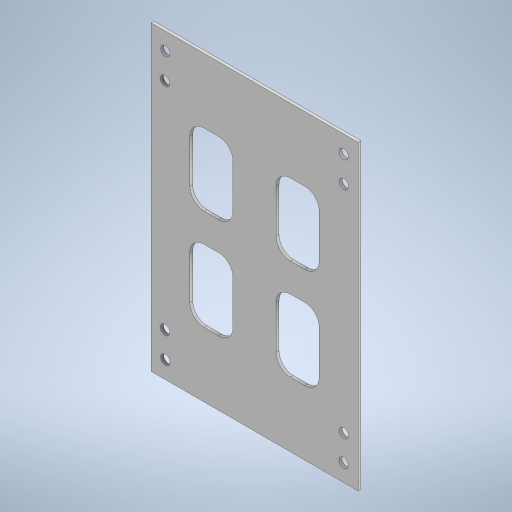
# Autodesk Inventor part: battery_box_24V_side1
Saved by Autodesk Inventor 2023 (Build 270158000, 158)
## iProperties
Created: 2023-05-28
Part Number: battery_box_24V_side1
Material: 一般
Document SubType Name: Sheet Metal
Designer: 310611102
Density: 1 g/cm^3
Sheet Metal Rule: Default_mm
Appearance: 預設
Author: 310611102
Autodesk Inventor part; units mm, degrees
ref_plane "YZ Plane" through (0, 0, 0) normal (1, 0, 0) x (0, 1, 0)
ref_plane "XZ Plane" through (0, 0, 0) normal (0, 1, 0) x (-1, 0, 0)
ref_plane "XY Plane" through (0, 0, 0) normal (0, 0, 1) x (1, 0, 0)
sketch "Sketch1" plane through (0, 0, 0) normal (0, 0, 1) x (1, 0, 0)
  line L0 (-36, 52.5) -> (36, 52.5)
  line L1 (36, 52.5) -> (36, -52.5)
  line L2 (36, -52.5) -> (-36, -52.5)
  line L3 (-36, -52.5) -> (-36, 52.5)
  line L4 (-36, 52.5) -> (36, -52.5) construction
  line L5 (36, 52.5) -> (-36, -52.5) construction
  circle A0 centre (31.1, -37.5) radius 1.6
  line L6 (0, 0) -> (12.8976, 0)
  line L7 (0, 0) -> (0, 11.3109)
  circle A1 centre (-31.1, -37.5) radius 1.6
  circle A2 centre (31.1, 37.5) radius 1.6
  circle A3 centre (-31.1, 37.5) radius 1.6
  circle A4 centre (-31, -46.5) radius 1.6
  circle A5 centre (-31, 46.5) radius 1.6
  circle A6 centre (31, -46.5) radius 1.6
  circle A7 centre (31, 46.5) radius 1.6
  dimension "d0" = 72
  dimension "d1" = 105
  dimension "d2" = 3.2
  dimension "d3" = 4.9
  dimension "d4" = 15
  dimension "d6" = 3.2
  dimension "d7" = 6
  dimension "d8" = 5
  measures "d0" distance of L1.end L2.end
  measures "d1" distance of L0.end L1.end
  measures "d2" diameter of A0
  measures "d3" distance from line of L1 A0.centre
  measures "d4" distance from line of L2 A0.centre
  measures "d6" diameter of A4
  measures "d7" distance from line of L2 A4.centre
  measures "d8" distance from line of L3 A4.centre
extrude "Plate1" add sketch "Sketch1" along normal blind 1
sketch "Sketch2" plane through (0, 0, 1) normal (0, 0, 1) x (1, 0, 0)
  line L0 (-17.5, 30) -> (-12.5, 30)
  line L1 (-7.5, 25) -> (-7.5, 10)
  line L2 (-12.5, 5) -> (-17.5, 5)
  line L3 (-22.5, 10) -> (-22.5, 25)
  line L4 (-22.5, 30) -> (-7.5, 5) construction
  line L5 (-7.5, 30) -> (-22.5, 5) construction
  line L6 (-28.3073, 0) -> (28.3073, 0)
  line L7 (0, 37.5) -> (0, -37.5)
  arc A0 (-17.5, 30) -> (-22.5, 25) centre (-17.5, 25) ccw
  arc A1 (-7.5, 25) -> (-12.5, 30) centre (-12.5, 25) ccw
  arc A2 (-12.5, 5) -> (-7.5, 10) centre (-12.5, 10) ccw
  arc A3 (-22.5, 10) -> (-17.5, 5) centre (-17.5, 10) ccw
  line L8 (17.5, 30) -> (12.5, 30)
  line L9 (7.5, 25) -> (7.5, 10)
  line L10 (12.5, 5) -> (17.5, 5)
  line L11 (22.5, 10) -> (22.5, 25)
  line L12 (22.5, 30) -> (7.5, 5) construction
  line L13 (7.5, 30) -> (22.5, 5) construction
  arc A4 (22.5, 25) -> (17.5, 30) centre (17.5, 25) ccw
  arc A5 (12.5, 30) -> (7.5, 25) centre (12.5, 25) ccw
  arc A6 (7.5, 10) -> (12.5, 5) centre (12.5, 10) ccw
  arc A7 (17.5, 5) -> (22.5, 10) centre (17.5, 10) ccw
  line L14 (-17.5, -30) -> (-12.5, -30)
  line L15 (-7.5, -25) -> (-7.5, -10)
  line L16 (-12.5, -5) -> (-17.5, -5)
  line L17 (-22.5, -10) -> (-22.5, -25)
  line L18 (-22.5, -30) -> (-7.5, -5) construction
  line L19 (-7.5, -30) -> (-22.5, -5) construction
  arc A8 (-22.5, -25) -> (-17.5, -30) centre (-17.5, -25) ccw
  arc A9 (-12.5, -30) -> (-7.5, -25) centre (-12.5, -25) ccw
  arc A10 (-7.5, -10) -> (-12.5, -5) centre (-12.5, -10) ccw
  arc A11 (-17.5, -5) -> (-22.5, -10) centre (-17.5, -10) ccw
  arc A12 (7.5, -25) -> (12.5, -30) centre (12.5, -25) ccw
  line L20 (7.5, -25) -> (7.5, -10)
  line L21 (17.5, -30) -> (12.5, -30)
  arc A13 (17.5, -30) -> (22.5, -25) centre (17.5, -25) ccw
  arc A14 (12.5, -5) -> (7.5, -10) centre (12.5, -10) ccw
  line L22 (22.5, -10) -> (22.5, -25)
  arc A15 (22.5, -10) -> (17.5, -5) centre (17.5, -10) ccw
  line L23 (7.5, -30) -> (22.5, -5) construction
  line L24 (22.5, -30) -> (7.5, -5) construction
  line L25 (12.5, -5) -> (17.5, -5)
  point P0 (0, 0)
  point P1 (-15, 17.5)
  point P2 (0, 0)
  point P3 (15, 17.5)
  point P4 (-15, -17.5)
  point P5 (15, -17.5)
  dimension "d9" = 15
  dimension "d10" = 25
  dimension "d12" = 10
  dimension "d13" = 15
  dimension "d14" = 5
  constraints: 52 end point, 51 symmetric about line, 32 point on circle, 32 point on line, 16 centre point, 8 tangent, 4 midpoint, 3 equal radius, 2 horizontal, 2 parallel, 1 coincident, 1 perpendicular, 1 vertical, 12 other
  measures "d9" distance of L4.start L5.start
  measures "d10" distance of L5.start L4.end
  measures "d12" diameter of L2 L6
  measures "d13" diameter of L1 L7
  measures "d14" radius of A0
extrude "Cut1" cut sketch "Sketch2" against normal blind 1
equation "\"d15\" = 厚度"
equation "\"d5\" = 厚度"
equation "\"折彎半徑\" = 厚度"
equation "\"折彎離隙寬度\" = 厚度"
equation "\"折彎離隙深度\" = 0.5 * 厚度"
equation "\"轉角離隙大小\" = 4 * 厚度"
equation "\"最小剩餘\" = 2 * 厚度"
equation "\"轉移半徑\" = 折彎半徑"
equation "\"Jacobi半徑大小\" = 折彎半徑"
equation "\"間隙大小\" = 厚度"
equation "\"厚度\" = 1"
body "Solid1"
